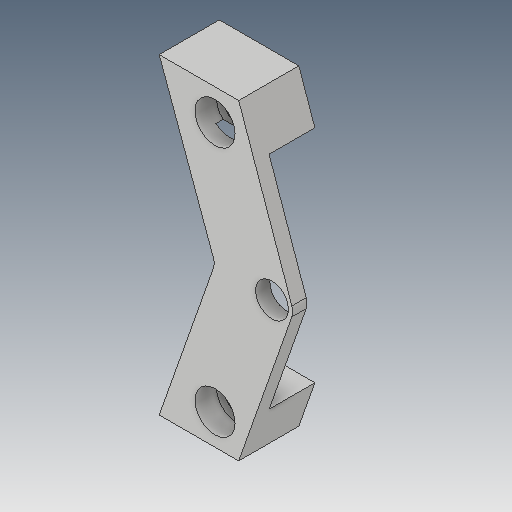
# Autodesk Inventor part: 20_focus_inlet_plate_top
Saved by Autodesk Inventor 2019.4 (Build 234330000, 330)
## iProperties
Created: 2020-02-05
Part Number: 20_focus_inlet_plate_top
Material: Generic
Document SubType Name: Modeling
Designer: marsikovabarbora
Density: 1 g/cm^3
Appearance: Default
Author: marsikovabarbora
Autodesk Inventor part; units mm, degrees
ref_plane "YZ Plane" through (0, 0, 0) normal (1, 0, 0) x (0, 1, 0)
ref_plane "XZ Plane" through (0, 0, 0) normal (0, 1, 0) x (-1, 0, 0)
ref_plane "XY Plane" through (0, 0, 0) normal (0, 0, 1) x (1, 0, 0)
sketch "Sketch1" plane through (0, 0, 0) normal (0, 0, 1) x (1, 0, 0)
  circle A0 centre (1.9608, 0) radius 2 construction
  circle A1 centre (-6, -17.5) radius 1.5 construction
  circle A2 centre (-6, 17.5) radius 1.5 construction
  line L0 (11.3072, 21.8) -> (-13.8, 21.8) construction
  line L1 (-13.8, 21.8) -> (-13.8, -21.8) construction
  line L2 (-13.8, -21.8) -> (11.3072, -21.8) construction
  line L3 (11.3072, -21.8) -> (11.3072, 21.8) construction
  line L4 (-18.8214, 0) -> (16.3286, 0) construction
  line L5 (-2.5075, 14.4235) -> (-13.8, 14.4235) construction
  circle A3 centre (-6, -17.5) radius 1.5 construction
  line L6 (11.3072, -21.8) -> (-13.8, -21.8) construction
  line L7 (-13.8, -21.8) -> (11.3072, -21.8)
  line L8 (-2.5075, -14.4235) -> (-13.8, -14.4235) construction
  circle A4 centre (-6, 17.5) radius 1.6
  circle A5 centre (-6, -17.5) radius 1.6
  line L9 (-13.8, 21.8) -> (11.3072, 21.8)
  line L10 (11.3072, 21.8) -> (11.3072, 15.4235)
  line L11 (11.3072, 15.4235) -> (-13.8, 15.4235)
  line L12 (-13.8, 15.4235) -> (-13.8, 21.8)
  line L13 (11.3072, 21.8) -> (11.3072, -21.8) construction
  line L14 (-13.8, -21.8) -> (11.3072, -21.8)
  line L15 (11.3072, -21.8) -> (11.3072, -15.4235)
  line L16 (11.3072, -15.4235) -> (-13.8, -15.4235)
  line L17 (-13.8, -15.4235) -> (-13.8, -21.8)
  point P0 (0, 0)
  dimension "d0" = 0.1
  dimension "d1" = 0.1
  dimension "d13" = 1
  constraints: 24 end point, 9 symmetric about line, 3 centre point, 2 parallel, 2 point on line, 1 horizontal, 1 perpendicular, 1 other
  measures "d0" radial gap between concentric circles of A2 A4
  measures "d1" radial gap between concentric circles of A1 A5
  measures "d13" distance between parallel lines of L11 L5
extrude "Extrusion1" add sketch "Sketch1" along normal blind 6.4
sketch "Sketch2" plane through (0, 0, 6.4) normal (0, 0, 1) x (1, 0, 0)
  circle A0 centre (-6, 17.5) radius 1.6 construction
  circle A1 centre (-6, -17.5) radius 1.6 construction
  line L0 (11.3072, 21.8) -> (-13.8, 21.8) projected
  line L1 (-13.8, -21.8) -> (11.3072, -21.8) projected
  line L2 (-13.8, 21.8) -> (11.3072, 21.8)
  line L3 (11.3072, 21.8) -> (11.3072, -21.8)
  line L4 (11.3072, -21.8) -> (-13.8, -21.8)
  line L5 (-13.8, -21.8) -> (-13.8, 21.8)
  circle A2 centre (-6, -17.5) radius 1.7
  circle A3 centre (-6, 17.5) radius 1.7
  circle A4 centre (1.9608, 0) radius 2 construction
  circle A5 centre (1.9608, 0) radius 2.3
  line L6 (-2.9164, -21.8) -> (3.0965, -2)
  line L7 (3.0965, 2) -> (-2.9164, 21.8)
  line L8 (-13.8, 21.8) -> (11.3072, 21.8) projected
  point P0 (0, 0)
  dimension "d6" = 0.1
  dimension "d7" = 0.1
  dimension "d8" = 0.3
  constraints: 12 end point, 3 centre point, 2 parallel, 2 point on circle, 2 point on line, 1 horizontal, 1 perpendicular
  measures "d6" radial gap between concentric circles of A1 A2
  measures "d7" radial gap between concentric circles of A0 A3
  measures "d8" radial gap between concentric circles of A4 A5
extrude "Extrusion2" add sketch "Sketch2" along normal blind 2 contours L3 L1 L6 A5 L7 L0 | L7 A5 L6 L1 L5 L0
sketch "Sketch3" plane through (0, 0, 8.4) normal (0, 0, 1) x (1, 0, 0)
  circle A0 centre (1.9608, 0) radius 2.3 construction
  circle A1 centre (-6, 17.5) radius 1.7 construction
  circle A2 centre (-6, -17.5) radius 1.7 construction
  line L0 (11.3072, 21.8) -> (-13.8, 21.8) construction
  line L1 (-13.8, 21.8) -> (-13.8, -21.8) construction
  line L2 (-13.8, -21.8) -> (11.3072, -21.8) construction
  line L3 (11.3072, -21.8) -> (11.3072, 21.8) construction
  circle A3 centre (-6, -17.5) radius 2.8
  circle A4 centre (-6, 17.5) radius 2.8
  point P0 (0, 0)
  dimension "d9" = 5.6
  dimension "d10" = 5.6
  constraints: 2 centre point, 2 coincident
  measures "d9" diameter of A3
  measures "d10" diameter of A4
extrude "Extrusion3" cut sketch "Sketch3" against normal blind 3
sketch "Sketch4" plane through (0, 0, 8.4) normal (0, 0, 1) x (1, 0, 0)
  circle A0 centre (-6, -17.5) radius 2.8 construction
  circle A1 centre (-6, 17.5) radius 2.8 construction
  circle A2 centre (1.9608, 0) radius 2.3 construction
  line L0 (11.3072, 21.8) -> (-13.8, 21.8) construction
  line L1 (-13.8, 21.8) -> (-13.8, -21.8) construction
  line L2 (-13.8, -21.8) -> (11.3072, -21.8) construction
  line L3 (11.3072, -21.8) -> (11.3072, 21.8) projected
  line L4 (11.3072, -21.8) -> (11.3072, 21.8) projected
  line L5 (11.3072, 21.8) -> (-2.6928, 21.8)
  line L6 (-13.8, 21.8) -> (11.3072, 21.8) projected
  line L7 (-2.6928, 21.8) -> (4.7397, 0.6635)
  line L8 (4.7397, -0.6635) -> (-2.6928, -21.8)
  line L9 (-13.8, -21.8) -> (11.3072, -21.8) projected
  line L10 (-2.6928, -21.8) -> (11.3072, -21.8)
  line L11 (11.3072, -21.8) -> (11.3072, 21.8)
  arc A3 (4.7397, -0.6635) -> (4.7397, 0.6635) centre (2.853, 0) ccw
  line L12 (-13.8, 21.8) -> (-6.243, 1.0605)
  line L13 (-6.2354, -0.2877) -> (-13.8, -21.8)
  line L14 (-13.8, 21.8) -> (-13.8, -21.8)
  arc A4 (-6.2354, -0.2877) -> (-6.243, 1.0605) centre (-8.1221, 0.3758) ccw
  point P0 (4.973, 0)
  dimension "d14" = 14
  dimension "d17" = 2
  dimension "d18" = 2
  constraints: 16 end point, 4 point on circle, 4 point on line, 4 tangent, 2 centre point, 1 collinear, 1 horizontal, 1 parallel, 1 perpendicular
  measures "d14" distance of L0.start L5.end
  measures "d17" radius of A3
  measures "d18" radius of A4
extrude "Extrusion4" cut sketch "Sketch4" against normal through all contours L9 L8 A3 L7 L5 L3 | L14 L12 A4 L13
equation "\"d10\" = d9"
body "Solid1"
